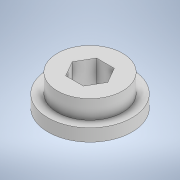
# Autodesk Inventor part: Hex Shaft Holder
Saved by Autodesk Inventor 2020 (Build 240168000, 168)
## iProperties
Created: 2020-01-18
Part Number: Hex Shaft Holder
Material: Generic
Document SubType Name: Modeling
Designer: kwruff
Density: 1 g/cm^3
Appearance: Default
Author: kwruff
Autodesk Inventor part; units mm, degrees
ref_plane "YZ Plane" through (0, 0, 0) normal (1, 0, 0) x (0, 1, 0)
ref_plane "XZ Plane" through (0, 0, 0) normal (0, 1, 0) x (-1, 0, 0)
ref_plane "XY Plane" through (0, 0, 0) normal (0, 0, 1) x (1, 0, 0)
sketch "Sketch1" plane through (0, 0, 0) normal (0, 1, 0) x (-1, 0, 0)
  circle A0 centre (0, 0) radius 17.145
  dimension "d0" = 34.29
  constraints: 1 centre point, 1 coincident
  measures "d0" diameter of A0
extrude "Extrusion1" add sketch "Sketch1" along normal blind 5.08
sketch "Sketch2" plane through (0, 5.08, 0) normal (0, 1, 0) x (1, 0, 0)
  circle A0 centre (0, 0) radius 13.335
  dimension "d3" = 26.67
  constraints: 1 centre point, 1 coincident
  measures "d3" diameter of A0
extrude "Extrusion2" add sketch "Sketch2" along normal blind 7.62
sketch "Sketch3" plane through (0, 12.7, 0) normal (0, 1, 0) x (1, 0, 0)
  line L0 (-3.6383, -6.3018) -> (-7.2767, 0)
  line L1 (-7.2767, 0) -> (-3.6383, 6.3018)
  line L2 (-3.6383, 6.3018) -> (3.6383, 6.3018)
  line L3 (3.6383, 6.3018) -> (7.2767, 0)
  line L4 (7.2767, 0) -> (3.6383, -6.3018)
  line L5 (3.6383, -6.3018) -> (-3.6383, -6.3018)
  point P0 (0, 0)
  point P1 (0, 0)
  constraints: 12 end point, 1 coincident, 13 other
extrude "Extrusion3" cut sketch "Sketch3" against normal blind 12.7
body "Solid1"
